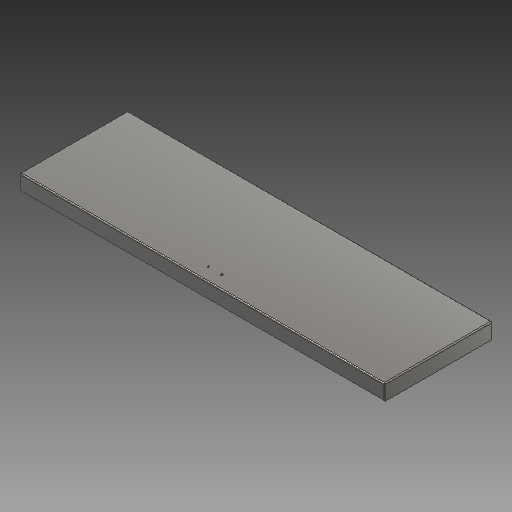
# Autodesk Inventor part: Base Gabinete
Saved by Autodesk Inventor 2017 (Build 210142000, 142)
## iProperties
Created: 2019-06-18
Part Number: Base Gabinete
Material: Stainless Steel
Description: Chapa de Aço Inox Aisi 304 - #1,5mm
Document SubType Name: Sheet Metal
Designer: leonardo.prado
Mass: 4380.63 g
Surface Area: 7342.98 cm^2
Volume: 547.578 cm^3
Density: 8 g/cm^3
Flat Pattern Width: 36.7871 cm
Flat Pattern Length: 101.138 cm
Flat Pattern Area: 3720.58 cm^2
Sheet Metal Rule: Default_mm
Sheet Metal Width: 367,871 mm
Sheet Metal Length: 1011,384 mm
Sheet Metal Area: 372058,461 mm^2
Appearance: Semi-Polished
Author: leonardo.prado
Comments: 1011 x 368
Autodesk Inventor part; units mm, degrees
note: some values were not read from the file. Chosen so that the rebuilt part matches the saved one: corner form of "Plate2".
ref_plane "YZ Plane" through (0, 0, 0) normal (1, 0, 0) x (0, 1, 0)
ref_plane "XZ Plane" through (0, 0, 0) normal (0, 1, 0) x (-1, 0, 0)
ref_plane "XY Plane" through (0, 0, 0) normal (0, 0, 1) x (1, 0, 0)
sketch "Sketch1" plane through (0, 0, 0) normal (0, 0, 1) x (1, 0, 0)
  line L0 (468.299, -139.1495) -> (-468.299, -139.1495)
  line L1 (-468.299, -139.1495) -> (-468.299, 139.1495)
  line L2 (-468.299, 139.1495) -> (468.299, 139.1495)
  line L3 (468.299, 139.1495) -> (468.299, -139.1495)
  line L4 (468.299, -139.1495) -> (-468.299, 139.1495) construction
  line L5 (-468.299, -139.1495) -> (468.299, 139.1495) construction
  point P0 (0, 0)
  dimension "d0" = 936.598
  dimension "d1" = 278.299
  measures "d0" distance of L1.end L2.end
  measures "d1" distance of L0.end L1.end
extrude "Plate1" add sketch "Sketch1" along normal blind 1.5
sketch "Sketch2" plane through (-468.299, -137.6495, 1.5) normal (0, -1, 0) x (1, 0, 0)
  line L0 (936.598, 0) -> (0, 0)
  line L1 (0, 0) -> (0, -40)
  line L2 (0, -40) -> (936.598, -40)
  line L3 (936.598, -40) -> (936.598, 0)
  constraints: 6 end point, 1 horizontal, 1 perpendicular, 1 vertical
edge flange "Flange1" height 40 angle 90 thickness 1.5 bend radius 1.5 thickness toward (0, -1, 0) relief tear relief width 1.5 relief depth 0.75 corner gap 1.5 corner form 2 edges at (0, -139.1495, 0) (-468.299, 0, 0) (0, 139.1495, 0) (468.299, 0, 0) wall of the first edge with corners at (468.299, -137.6495, 1.5) (-468.299, -137.6495, 1.5) (-468.299, -137.6495, -38.5) (468.299, -137.6495, -38.5)
bend "Bend1"
corner "Corner1"
sketch "Sketch3" plane through (-465.7383, -139.1495, -37) normal (0, 0, -1) x (-1, 0, 0)
  line L0 (-931.4767, 0) -> (0, 0)
  line L1 (0, 0) -> (0, 10)
  line L2 (0, 10) -> (-931.4767, 10)
  line L3 (-931.4767, 10) -> (-931.4767, 0)
  constraints: 6 end point, 1 horizontal, 1 perpendicular, 1 vertical
edge flange "Flange2" height 10 angle 90 thickness 1.5 bend radius 1.5 thickness toward (0, 0, -1) relief tear relief width 1.5 relief depth 0.75 corner gap 1.5 corner form 0 edges at (0, -137.6495, -38.5) (0, 137.6495, -38.5) wall of the first edge with corners at (465.7383, -139.1495, -37) (-465.7383, -139.1495, -37) (-465.7383, -129.1495, -37) (465.7383, -129.1495, -37)
bend "Bend2"
corner "Corner2"
sketch "Sketch4" plane through (0, 0, 1.5) normal (0, 0, 1) x (1, 0, 0)
  circle A0 centre (17.5, -104.6495) radius 2.25 projected
  circle A1 centre (-17.5, -104.6495) radius 2.25 projected
  point P0 (0, 0)
extrude "Extrusion1" cut sketch "Sketch4" against normal through all
equation "\"d3\" = BendReliefWidth"
equation "\"d4\" = BendReliefDepth"
equation "\"d5\" = MinimumRemnant"
equation "\"d6\" = BendRadius"
equation "\"d9\" = BendRadius"
equation "\"d10\" = CornerReliefSize"
equation "\"d11\" = GapSize"
equation "\"d12\" = JacobiRadiusSize"
equation "\"d13\" = BendReliefWidth"
equation "\"d14\" = BendReliefDepth"
equation "\"d15\" = MinimumRemnant"
equation "\"d16\" = BendRadius"
equation "\"d19\" = BendRadius"
equation "\"d20\" = CornerReliefSize"
equation "\"d21\" = GapSize"
equation "\"d22\" = JacobiRadiusSize"
equation "\"BendRadius\" = Thickness"
equation "\"BendReliefWidth\" = Thickness"
equation "\"BendReliefDepth\" = 0.5 * Thickness"
equation "\"CornerReliefSize\" = 4 * Thickness"
equation "\"MinimumRemnant\" = 2 * Thickness"
equation "\"TransitionRadius\" = BendRadius"
equation "\"JacobiRadiusSize\" = BendRadius"
equation "\"GapSize\" = Thickness"
equation "\"d2\" = BendRadius"
equation "\"Thickness\" = 1.5"
body "Solid1"
